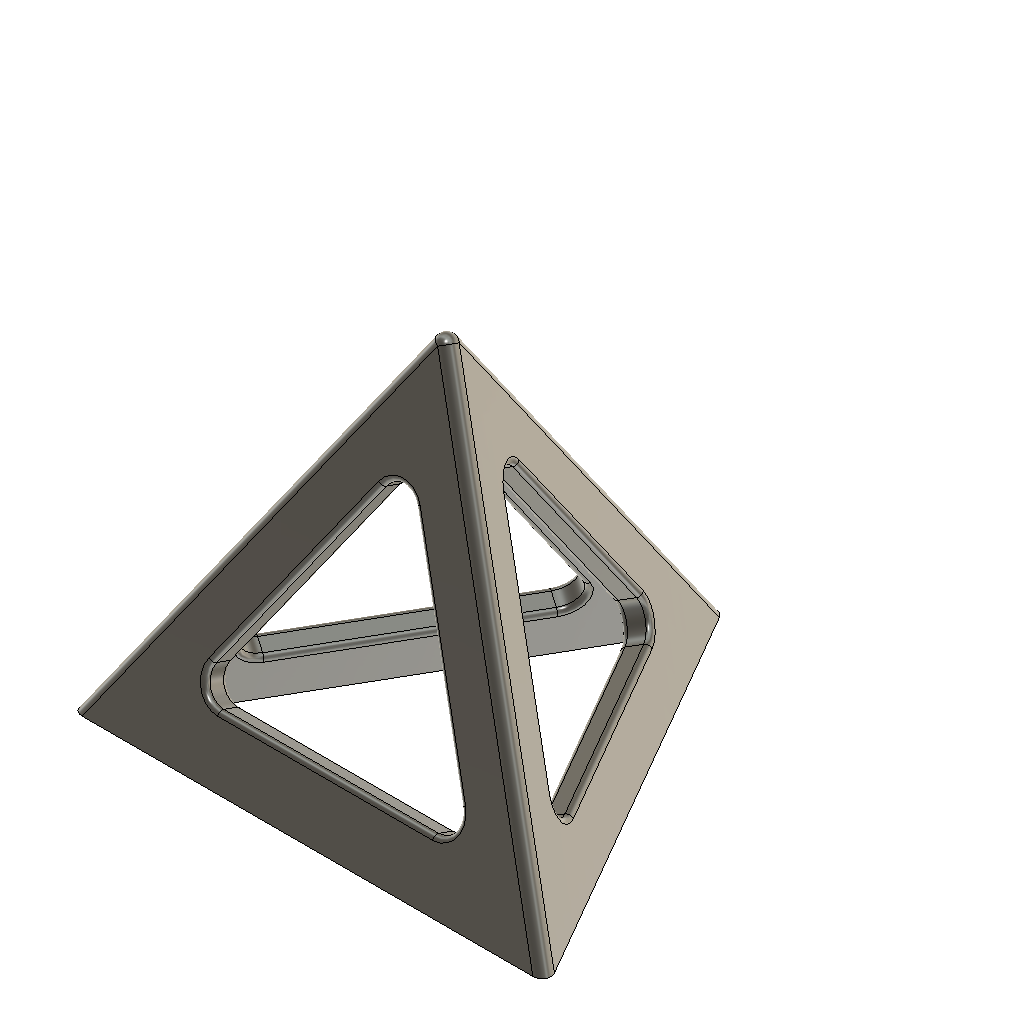
Painters Tripod (Autodesk Fusion 360 design; units mm, degrees)
part number: 2026-09-29-23-51-31-468
Autodesk Fusion 360 part; units mm, degrees
sketch "Triangle" plane through (0, 0, 0) normal (0, 0, 1) x (1, 0, 0)
  line L0 (-25, -14.4338) -> (25, -14.4338)
  line L1 (25, -14.4338) -> (0, 28.8675)
  line L2 (0, 28.8675) -> (-25, -14.4338)
  line L3 (0, -14.4338) -> (0, 28.8675) construction
  line L4 (25, -14.4338) -> (-12.5, 7.2169) construction
  dimension "d1" = 50
  constraint equal L0 L2
  constraint equal L0 L1
  constraint midpoint L0 L3.start
  constraint midpoint L2 L4.end
  constraint coincident L3 origin
  constraint coincident L4 origin
  constraint horizontal L0
  measures "d1" distance of L0.start L0.end
ref_plane "WorkPlane1" through (0, 0, 40.8248) normal (0, 0, 1) x (1, 0, 0)
sketch "Loft Point" plane through (0, 0, 40.8248) normal (0, 0, 1) x (1, 0, 0)
loft "Loft1" add profiles "Triangle" section 1 section 2 point at (0, 0, 40.8248)
shell "Shell1" thickness 2.5 removed faces 1 at (0, 0, 0)
sketch "Sketch3" plane through (0, -12.83, 4.5361) normal (0, -0.942809, 0.333333) x (1, 0, 0)
  line L0 (-25, -4.8113) -> (25, -4.8113)
  line L1 (25, -4.8113) -> (0, 38.49)
  line L2 (0, 38.49) -> (-25, -4.8113)
  line L3 (-14.6077, 1.1887) -> (14.6077, 1.1887)
  line L4 (14.6077, 1.1887) -> (0, 26.49)
  line L5 (0, 26.49) -> (-14.6077, 1.1887)
  dimension "d5" = -6
extrude "Extrude1" cut sketch "Sketch3" against normal up to surface (2.5 mm away) contours L3 L4 L5
pattern_circular "C-Pattern1" count 3 over 360 about axis through (0, 0, 1.75) along (0, 0, 1) of "Extrude1"
fillet "Fillet1" radius 1 3 edges at (-12.5, -7.2169, 20.4124) (12.5, -7.2169, 20.4124) (0, 14.4338, 20.4124)
fillet "Fillet1" radius 2 9 edges at (-14.6077, -11.2552, 5.2402) (0, -2.8215, 29.0945) (14.6077, -11.2552, 5.2402) (17.0512, -7.023, 5.2402) (2.4435, 18.2783, 5.2402) (2.4435, 1.4107, 29.0945) (-2.4435, 1.4107, 29.0945) (-2.4435, 18.2783, 5.2402) (-17.0512, -7.023, 5.2402)
fillet "Fillet1" radius 0.5 18 edges at (-10.7679, -2.2169, 17.584) (-8.7267, -3.3954, 16.7507) (-10.7679, 6.2169, 5.6569) (-8.7267, 5.0384, 4.8235) (-1.4229, 9.2552, 16.7507) (-3.4641, 10.4338, 17.584) (8.7267, 5.0384, 4.8235) (10.7679, 6.2169, 5.6569) (-7.3038, -8.2169, 17.584) (-7.3038, -5.8599, 16.7507) (0, -10.0767, 4.8235) (0, -12.4338, 5.6569) (7.3038, -8.2169, 17.584) (7.3038, -5.8599, 16.7507) (10.7679, -2.2169, 17.584) (8.7267, -3.3954, 16.7507) (3.4641, 10.4338, 17.584) (1.4229, 9.2552, 16.7507)
equation "d2 = ( d1 * sqrt(6) ) / 3"
